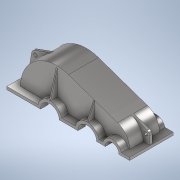
# Autodesk Inventor part: МПСТ Крышка корпуса
Saved by Autodesk Inventor 2022.1 (Build 261234020, 234B)
## iProperties
Created: 2021-12-09
Part Number: МПСТ Крышка корпуса
Material: Сталь, углеродистая
Document SubType Name: Modeling
Designer: Алексанян Г.
Density: 7.85 g/cm^3
Appearance: С умеренной полировкой
Author: Алексанян Г.
Autodesk Inventor part; units mm, degrees
ref_plane "XZ Plane" through (0, 0, 0) normal (0, 1, 0) x (-1, 0, 0)
ref_plane "XY Plane" through (0, 0, 0) normal (0, 0, 1) x (1, 0, 0)
sketch "Эскиз1" plane through (0, 0, 0) normal (0, 1, 0) x (-1, 0, 0)
  line L0 (493, -175) -> (-493, -175)
  line L1 (-493, -175) -> (-493, 175)
  line L2 (-493, 175) -> (493, 175)
  line L3 (493, 175) -> (493, -175)
  line L4 (493, -175) -> (-493, 175) construction
  line L5 (-493, -175) -> (493, 175) construction
  point P0 (0, 0)
  dimension "d0" = 350
  dimension "d1" = 986
  constraints: 12 end point, 2 midpoint, 2 parallel, 1 horizontal, 1 perpendicular
  measures "d0" distance of L0.end L1.end
  measures "d1" distance of L0.start L0.end
extrude "Выдавливание1" add sketch "Эскиз1" along normal blind 22.5
sketch "Эскиз2" plane through (0, 0, 0) normal (0, 0, 1) x (1, 0, 0)
  line L0 (493, 22.5) -> (-493, 22.5) projected
  arc A0 (-52.6766, 296.3858) -> (-438, 22.5) centre (-148, 22.5) ccw
  line L1 (-52.6766, 296.3858) -> (340.7917, 159.4429)
  arc A1 (438.13, 22.5) -> (340.7917, 159.4429) centre (293.13, 22.5) ccw
  point P0 (0, 0)
  dimension "d4" = 290
  dimension "d5" = 145
  dimension "d7" = 55
  dimension "d69" = 876.13
  constraints: 4 point on circle, 4 point on line, 2 centre point, 2 end point, 2 tangent
  measures "d4" radius of A0
  measures "d5" radius of A1
  measures "d7" distance of L0.end A0.end
  measures "d69" distance of A1.start A0.end
extrude "Выдавливание2" add sketch "Эскиз2" along normal mid plane 240
shell "Оболочка1" thickness 6 removed faces 1 at (-164.3333, 0, 58.3333)
sketch "Эскиз3" plane through (-487, 16.5, 169) normal (0, -1, 0) x (1, 0, 0)
  line L0 (55.0634, -283) -> (919.0004, -283) projected
  line L1 (55.0634, -55) -> (55.0634, -283) projected
  line L2 (919.0004, -55) -> (55.0634, -55) projected
  line L3 (919.0004, -283) -> (919.0004, -55) projected
  line L4 (0, 0) -> (974, 0) projected
  line L5 (0, -338) -> (0, 0) projected
  line L6 (974, -338) -> (0, -338) projected
  line L7 (974, 0) -> (974, -338) projected
  point P0 (487, -169)
extrude "Выдавливание3" add sketch "Эскиз3" along normal up to surface (16.5 mm away)
sketch "Эскиз4" plane through (-493, 0, 175) normal (0, 0, 1) x (1, 0, 0)
  line L0 (0, 0) -> (986, 0) projected
  circle A0 centre (846, 0) radius 55
  circle A1 centre (646, 0) radius 75
  circle A2 centre (346, 0) radius 75
  circle A3 centre (346, 0) radius 97.5
  circle A4 centre (646, 0) radius 97.5
  circle A5 centre (846, 0) radius 77.5
  point P0 (493, 0)
  point P1 (493, 0)
  point P2 (923.5, 0)
  point P3 (768.5, 0)
  point P4 (791, 0)
  point P5 (901, 0)
  point P6 (743.5, 0)
  point P7 (548.5, 0)
  point P8 (571, 0)
  point P9 (721, 0)
  point P10 (443.5, 0)
  point P11 (248.5, 0)
  point P12 (271, 0)
  point P13 (421, 0)
  dimension "d13" = 140
  dimension "d14" = 200
  dimension "d15" = 300
  dimension "d16" = 110
  dimension "d17" = 150
  dimension "d18" = 150
  dimension "d19" = 22.5
  dimension "d20" = 22.5
  dimension "d21" = 22.5
  constraints: 6 centre point, 3 coincident, 3 horizontal alignment, 1 midpoint
  measures "d13" distance of L0.end point (846, 0)
  measures "d14" distance of point (646, 0) point (846, 0)
  measures "d15" distance of point (346, 0) point (646, 0)
  measures "d16" diameter of A0
  measures "d17" diameter of A1
  measures "d18" diameter of A2
  measures "d19" radial gap between concentric circles of A2 A3
  measures "d20" radial gap between concentric circles of A1 A4
  measures "d21" radial gap between concentric circles of A0 A5
extrude "Выдавливание4" add sketch "Эскиз4" against normal up to surface (55 mm away) contours A2 L0 A3 | A1 L0 A4 | A0 L0 A5 picked at (256.3308, 4.6252) picked at (556.3308, 4.6252) picked at (810.9156, 60.3286)
extrude "Выдавливание5" cut sketch "Эскиз4" against normal up to surface (61 mm away) contours L0 A2 | L0 A1 | L0 A0 picked at (362.7619, 29.314) picked at (666.2254, 14.6946) picked at (861.8995, 13.02)
sketch "Эскиз5" plane through (493, 0, -175) normal (0, 0, -1) x (-1, 0, 0)
  line L0 (0, 0) -> (986, 0) projected
  circle A0 centre (140, 0) radius 55
  circle A1 centre (340, 0) radius 75
  circle A2 centre (640, 0) radius 75
  circle A3 centre (140, 0) radius 77.5
  circle A4 centre (340, 0) radius 97.5
  circle A5 centre (640, 0) radius 97.5
  point P0 (493, 0)
  point P1 (493, 0)
  point P2 (737.5, 0)
  point P3 (542.5, 0)
  point P4 (565, 0)
  point P5 (715, 0)
  point P6 (437.5, 0)
  point P7 (242.5, 0)
  point P8 (265, 0)
  point P9 (415, 0)
  point P10 (217.5, 0)
  point P11 (62.5, 0)
  point P12 (85, 0)
  point P13 (195, 0)
  dimension "d26" = 140
  dimension "d27" = 200
  dimension "d28" = 300
  dimension "d29" = 110
  dimension "d30" = 150
  dimension "d31" = 150
  dimension "d32" = 22.5
  dimension "d33" = 22.5
  dimension "d34" = 22.5
  constraints: 6 centre point, 3 coincident, 3 horizontal alignment, 1 midpoint
  measures "d26" distance of L0.start point (140, 0)
  measures "d27" distance of point (140, 0) point (340, 0)
  measures "d28" distance of point (340, 0) point (640, 0)
  measures "d29" diameter of A0
  measures "d30" diameter of A1
  measures "d31" diameter of A2
  measures "d32" radial gap between concentric circles of A0 A3
  measures "d33" radial gap between concentric circles of A1 A4
  measures "d34" radial gap between concentric circles of A2 A5
extrude "Выдавливание6" add sketch "Эскиз5" against normal up to surface (55 mm away) contours A0 L0 A3 | A1 L0 A4 | A2 L0 A5 picked at (104.9156, 60.3286) picked at (250.3308, 4.6252) picked at (550.3308, 4.6252)
extrude "Выдавливание7" cut sketch "Эскиз5" against normal up to surface (61 mm away) contours L0 A0 | L0 A1 | L0 A2 picked at (153.5485, 12.3511) picked at (356.7619, 29.314) picked at (660.2254, 14.6946)
sketch "Эскиз6" plane through (0, 0, 0) normal (0, 0, 1) x (1, 0, 0)
  line L0 (493, 22.5) -> (427.162, 22.5) projected
  line L1 (488, 22.5) -> (488, 86.8846)
  line L2 (-52.6766, 296.3858) -> (340.7917, 159.4429) projected
  line L3 (340.7917, 159.4429) -> (467.861, 115.2176)
  arc A0 (488, 86.8846) -> (467.861, 115.2176) centre (458, 86.8846) ccw
  arc A1 (438.13, 22.5) -> (340.7917, 159.4429) centre (293.13, 22.5) ccw projected
  line L4 (-241.8683, 22.5) -> (-493, 22.5) projected
  line L5 (-488, 22.5) -> (-457.5055, 195.4426)
  arc A2 (-52.6766, 296.3858) -> (-438, 22.5) centre (-148, 22.5) ccw projected
  line L6 (-493, 0) -> (-493, 22.5) projected
  line L7 (-438.2219, 218.424) -> (-302.8556, 267.6933)
  arc A3 (-438.2219, 218.424) -> (-457.5055, 195.4426) centre (-427.9613, 190.2332) ccw
  circle A4 centre (-427.9613, 190.2332) radius 15
  circle A5 centre (458, 86.8846) radius 15
  line L8 (427.162, 22.5) -> (438.13, 22.5) projected
  point P0 (0, 0)
  point P1 (-454.4979, 212.5)
  dimension "d39" = 5
  dimension "d40" = 30
  dimension "d41" = 5
  dimension "d42" = 80
  dimension "d44" = 190
  dimension "d45" = 120
  dimension "d46" = 30
  dimension "d47" = 30
  dimension "d48" = 30
  constraints: 8 end point, 5 point on circle, 4 centre point, 4 point on line, 4 tangent, 2 coincident, 1 collinear, 1 vertical
  measures "d39" distance from line of L0.start L1
  measures "d40" radius of A0
  measures "d41" distance from line of L6 L5.start
  measures "d42" angle of L4 L5
  measures "d44" vertical distance of L5.start point (-454.498, 212.5)
  measures "d45" angle of L5 L7
  measures "d46" radius of A3
  measures "d47" diameter of A4
  measures "d48" diameter of A5
extrude "Выдавливание8" add sketch "Эскиз6" along normal mid plane 20
sketch "Эскиз7" plane through (-493, 0, 175) normal (0, 0, 1) x (1, 0, 0)
  arc A0 (421, 0) -> (271, 0) centre (346, 0) ccw projected
  arc A1 (721, 0) -> (571, 0) centre (646, 0) ccw projected
  point P0 (493, 0)
  constraints: 2 coincident
ref_plane "РабПлоскость2" through (153, 0, 175) normal (1, 0, 0) x (0, 1, 0)
ref_plane "РабПлоскость1" through (-147, 0, 175) normal (1, 0, 0) x (0, 1, 0)
ref_plane "РабПлоскость3" through (-147, 0, 175) normal (1, 0, 0) x (0, 1, 0)
ref_plane "РабПлоскость4" through (153, 0, 175) normal (1, 0, 0) x (0, 1, 0)
sketch "Эскиз8" plane through (-147, 0, 175) normal (1, 0, 0) x (0, 1, 0)
  line L0 (97.5, 0) -> (97.5, -55) projected
  line L1 (97.5, -0.7774) -> (296.3858, -55)
  line L2 (312.5, -55) -> (22.5, -55) projected
  point P0 (0, -175)
  constraints: 2 end point, 1 point on line
extrude "Ребро жесткости2" add sketch "Эскиз8" along normal mid plane 10 rib yes fills toward (196.9298, -27.9369) open curves L1
mirror "Зеркальное отражение1" about plane through (0, 0, 0) normal (0, 0, 1) of "Ребро жесткости2"
sketch "Эскиз11" plane through (153, 0, 175) normal (1, 0, 0) x (0, 1, 0)
  line L0 (97.5, -350) -> (97.5, -295) projected
  line L1 (97.5, -350) -> (219.5597, -295)
  line L2 (296.3858, -295) -> (159.4429, -295) projected
  line L3 (296.3858, -55) -> (296.3858, -295) projected
  line L4 (97.3717, -295) -> (22.5, -295) projected
  line L5 (296.3858, -295) -> (22.5, -295)
  point P0 (0, -175)
  constraints: 4 end point, 1 collinear, 1 point on line
extrude "Ребро жесткости3" add sketch "Эскиз11" along normal mid plane 10 rib yes fills toward (97.55, -322.5) open curves L0 L1
mirror "Зеркальное отражение2" about plane through (0, 0, 0) normal (0, 0, 1) of "Ребро жесткости3"
